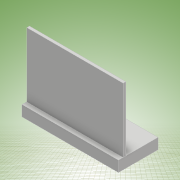
# Autodesk Inventor part: Wall_desk
Saved by Autodesk Inventor 2017 (Build 210142000, 142)
## iProperties
Created: 2018-06-04
Part Number: Wall_desk
Material: Generic
Document SubType Name: Modeling
Designer: Spark Electronics
Density: 1 g/cm^3
Appearance: Default
Author: Spark Electronics
Autodesk Inventor part; units mm, degrees
ref_plane "YZ Plane" through (0, 0, 0) normal (1, 0, 0) x (0, 1, 0)
ref_plane "XZ Plane" through (0, 0, 0) normal (0, 1, 0) x (-1, 0, 0)
ref_plane "XY Plane" through (0, 0, 0) normal (0, 0, 1) x (1, 0, 0)
sketch "Sketch1" plane through (0, 0, 0) normal (0, 0, 1) x (1, 0, 0)
  line L0 (457.2, -187.511) -> (-457.2, -187.511)
  line L1 (-457.2, -187.511) -> (-457.2, 187.511)
  line L2 (-457.2, 187.511) -> (457.2, 187.511)
  line L3 (457.2, 187.511) -> (457.2, -187.511)
  line L4 (457.2, -187.511) -> (-457.2, 187.511) construction
  line L5 (-457.2, -187.511) -> (457.2, 187.511) construction
  point P0 (0, 0)
  dimension "d0" = 914.4
  constraints: 12 end point, 2 midpoint, 2 parallel, 1 horizontal, 1 perpendicular
  measures "d0" distance of L1.end L2.end
extrude "Extrusion1" add sketch "Sketch1" along normal blind 101.6
sketch "Sketch2" plane through (0, 0, 101.6) normal (0, 0, 1) x (1, 0, 0)
  line L0 (-456.2172, -142.8082) -> (457.0856, -142.8082)
  line L1 (457.0856, -142.8082) -> (457.0856, -117.2983)
  line L2 (457.0856, -117.2983) -> (-456.2172, -117.2983)
  line L3 (-456.2172, -117.2983) -> (-456.2172, -142.8082)
  point P0 (0, 0)
  constraints: 8 end point, 2 parallel, 1 horizontal, 1 perpendicular
extrude "Extrusion2" add sketch "Sketch2" along normal blind 609.6
body "Solid1"
